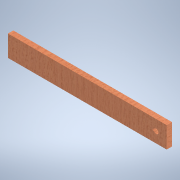
# Autodesk Inventor part: Hebel_camera
Saved by Autodesk Inventor 2021 (Build 250183000, 183)
## iProperties
Created: 2022-06-26
Part Number: Hebel_camera
Material: Holz (Eiche)
Document SubType Name: Modeling
Designer: adria
Density: 0.76 g/cm^3
Appearance: Weißeiche - natur - mittlerer Glanz
Mass: 90.6642 g
Surface Area: 309.732 cm^2
Volume: 119.295 cm^3
Author: adria
Autodesk Inventor part; units mm, degrees
ref_plane "YZ Plane" through (0, 0, 0) normal (1, 0, 0) x (0, 1, 0)
ref_plane "XZ Plane" through (0, 0, 0) normal (0, 1, 0) x (-1, 0, 0)
ref_plane "XY Plane" through (0, 0, 0) normal (0, 0, 1) x (1, 0, 0)
sketch "Skizze1" plane through (0, 0, 0) normal (0, 0, 1) x (1, 0, 0)
  line L0 (0, 40) -> (-300, 40)
  line L1 (-300, 40) -> (-300, 0)
  line L2 (-300, 0) -> (0, 0)
  line L3 (0, 0) -> (0, 40)
  line L4 (-360, 0) -> (60, 0) projected
  line L5 (0, -8) -> (0, 48) projected
  dimension "d0" = 300
  dimension "d1" = 40
  constraints: 8 end point, 2 parallel, 2 point on line, 1 horizontal, 1 perpendicular
  measures "d0" distance between parallel lines of L1 L3
  measures "d1" distance between parallel lines of L2 L0
extrude "Extrusion1" add sketch "Skizze1" along normal blind 10
sketch "Skizze2" plane through (0, 0, 0) normal (0, 0, -1) x (-1, 0, 0)
  line L0 (0, 40) -> (300, 40) projected
  line L1 (0, 0) -> (0, 40) projected
  point P0 (20, 20)
  dimension "d4" = 20
  dimension "d5" = 20
  measures "d4" distance from line of L0 point (20, 20)
  measures "d5" distance from line of L1 point (20, 20)
hole "Bohrung1" at (-20, 20, 0) direction (0, 0, 1) diameter 9 end through all
sketch "Skizze3" plane through (0, 0, 0) normal (0, 0, -1) x (-1, 0, 0)
  circle A0 centre (20, 20) radius 4.5 projected
  line L0 (0, 40) -> (300, 40) projected
  line L1 (20, 20) -> (24.5, 20)
  circle A1 centre (24.5, 20) radius 2
  point P0 (24.0556, 18.05)
  point P1 (24.0556, 21.95)
  dimension "d13" = 4
  constraints: 2 end point, 1 centre point, 1 coincident, 1 parallel, 2 other
  measures "d13" diameter of A1
extrude "Extrusion2" cut sketch "Skizze3" against normal blind 10 contours A0 A1 picked at (25.084, 19.4875)
